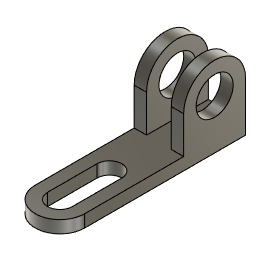
EX-05 (Autodesk Fusion 360 design; units mm, degrees)
Autodesk Fusion 360 part; units mm, degrees
sketch "Sketch1" plane through (0, 0, 0) normal (0, 0, 1) x (1, 0, 0)
  line L0 (-20, 0) -> (-150, 0)
  line L1 (-150, 0) -> (-150, 40)
  line L2 (-150, 40) -> (-20, 40)
  arc A0 (-20, 0) -> (-20, 40) centre (-20, 20) ccw
  arc A1 (-20, 10) -> (-20, 30) centre (-20, 20) ccw
  line L3 (-20, 10) -> (-60, 10)
  line L4 (-20, 30) -> (-60, 30)
  arc A2 (-60, 30) -> (-60, 10) centre (-60, 20) ccw
  dimension "d1" = 150
  dimension "d3" = 20
  dimension "d4" = 10
  dimension "d5" = 40
  dimension "d6" = 40
  dimension "d7" = 10
  constraint horizontal L0
  constraint vertical L1
  constraint horizontal L2
  constraint coincident L2 A0.end
  constraint coincident L0 A0.start
  constraint parallel L0 L3
  constraint horizontal L4
  constraint tangent L4 A2
  constraint tangent L3 A2
  constraint coincident A0 L0.start
  constraint coincident A0 L2.end
  measures "d1" distance of origin L0.end
  measures "d3" radius of A0
  measures "d4" radius of A1
  measures "d5" distance of A1.start L3.end
  measures "d6" distance of A1.end L4.end
  measures "d7" radius of A2
extrude "Extrude1" add sketch "Sketch1" along normal blind 10
move_body "Move1" bodies 1 to x (0, -1, 0) y (1, 0, 0) z (0, 0, 1) at (-150, -150, 0)
sketch "Sketch2" plane through (0, 0, 10) normal (0, 0, 1) x (-1, 0, 0)
  arc A0 (140, 130) -> (120, 130) centre (130, 130) ccw
  line L0 (140, 130) -> (140, 90)
  arc A1 (120, 90) -> (140, 90) centre (130, 90) ccw
  line L1 (120, 90) -> (120, 130)
  line L2 (150, 0) -> (150, 130)
  arc A2 (150, 130) -> (110, 130) centre (130, 130) ccw
  line L3 (110, 130) -> (110, 0)
  line L4 (110, 0) -> (150, 0)
  line L5 (140, 0) -> (140, 50)
  line L6 (140, 50) -> (150, 50)
  line L7 (110, 50) -> (120, 50)
  line L8 (120, 50) -> (120, 0)
  dimension "d10" = 50
  dimension "d11" = 10
  dimension "d12" = 10
  dimension "d13" = 50
  constraint coincident L4 L5.start
  constraint perpendicular L4 L5
  constraint perpendicular L2 L6
  constraint coincident L3 L7.start
  constraint perpendicular L3 L7
  constraint perpendicular L4 L8
  measures "d10" distance of L5.start L5.end
  measures "d11" distance of L5.end L6.end
  measures "d12" distance of L7.start L7.end
  measures "d13" distance of L7.end L8.end
extrude "Extrude2" add sketch "Sketch2" along normal blind 55 contours L2 L4 L5 L6 | L3 L4 L7 L8
sketch "Sketch3" plane through (-110, 0, 0) normal (1, 0, 0) x (0, 1, 0)
  line L0 (-130, 0) -> (0, 0)
  line L1 (0, 0) -> (0, 65)
  line L2 (0, 65) -> (-50, 65)
  line L3 (-50, 65) -> (-50, 10)
  line L4 (-50, 10) -> (-130, 10)
  line L5 (-130, 10) -> (-130, 0)
  arc A0 (0, 40) -> (-50, 40) centre (-25, 40) ccw
  circle A1 centre (-25, 40) radius 15
  dimension "d16" = 25
  dimension "d17" = 30
  constraint tangent L2 A0
  constraint coincident L1 A0.start
  constraint coincident L3 A0.end
  constraint concentric A0 A1
  measures "d16" radius of A0
  measures "d17" diameter of A1
extrude "Extrude3" cut sketch "Sketch3" against normal blind 10 contours L1 L2 A0 | L2 L3 A0 | A1
sketch "Sketch4" plane through (-150, 0, 0) normal (-1, 0, 0) x (0, -1, 0)
  line L0 (0, 0) -> (130, 0)
  line L1 (130, 0) -> (130, 10)
  line L2 (130, 10) -> (50, 10)
  line L3 (50, 10) -> (50, 65)
  line L4 (50, 65) -> (0, 65)
  line L5 (0, 65) -> (0, 0)
  arc A0 (50, 40) -> (0, 40) centre (25, 40) ccw
  circle A1 centre (25, 40) radius 15
  dimension "d20" = 25
  dimension "d21" = 30
  constraint tangent L4 A0
  constraint coincident L5 A0.end
  constraint concentric A0 A1
  measures "d20" radius of A0
  measures "d21" diameter of A1
extrude "Extrude4" cut sketch "Sketch4" against normal blind 10 contours L4 L5 A0 | L3 L4 A0 | A1
